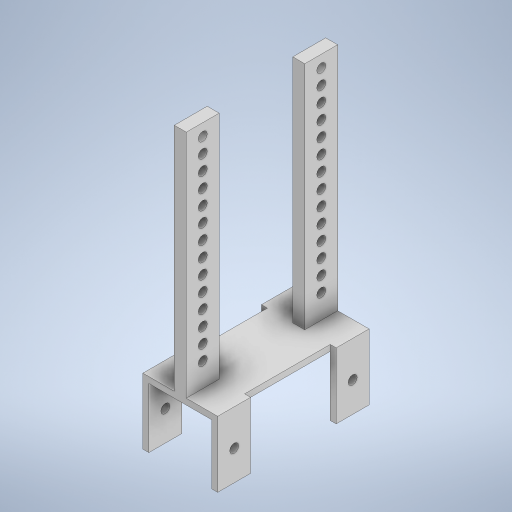
# Autodesk Inventor part: catcher_2ea
Saved by Autodesk Inventor 2024 (Build 280153000, 153)
## iProperties
Created: 2024-07-10
Part Number: catcher_2ea
Material: 일반
Document SubType Name: Modeling
Designer: Gihyeok Na
Density: 1 g/cm^3
Appearance: 기본값
Author: Gihyeok Na
Autodesk Inventor part; units mm, degrees
ref_plane "YZ Plane" through (0, 0, 0) normal (1, 0, 0) x (0, 1, 0)
ref_plane "XZ Plane" through (0, 0, 0) normal (0, 1, 0) x (-1, 0, 0)
ref_plane "XY Plane" through (0, 0, 0) normal (0, 0, 1) x (1, 0, 0)
sketch "스케치4" plane through (0, 0, 0) normal (0, 1, 0) x (-1, 0, 0)
  line L0 (-2, 5.5) -> (-2, -5.5)
  line L1 (-2, -5.5) -> (2, -5.5)
  line L2 (2, -5.5) -> (2, 5.5)
  line L3 (2, 5.5) -> (-2, 5.5)
  line L4 (-2, 5.5) -> (2, -5.5) construction
  line L5 (-2, -5.5) -> (2, 5.5) construction
  line L6 (15.7602, 19.8) -> (-23.0581, 19.8) construction
  line L7 (-2, 34.1) -> (-2, 45.1)
  line L8 (-2, 45.1) -> (2, 45.1)
  line L9 (2, 45.1) -> (2, 34.1)
  line L10 (2, 34.1) -> (-2, 34.1)
  line L11 (-2, 34.1) -> (2, 45.1) construction
  line L12 (-2, 45.1) -> (2, 34.1) construction
  point P0 (0, 0)
  point P1 (0, 0)
  point P2 (0, 39.6)
  point P3 (0, 39.6)
  dimension "d12" = 11
  dimension "d13" = 4
  dimension "d42" = 19.8
  constraints: 26 end point, 6 symmetric about line, 5 midpoint, 2 parallel, 1 horizontal, 1 perpendicular, 1 vertical
  measures "d12" distance of L0.start L0.end
  measures "d13" distance of L1.end L0.end
  measures "d42" distance from line of point (0, 0) L6
extrude "돌출3" add sketch "스케치4" along normal blind 77
sketch "스케치5" plane through (0, 0, 0) normal (0, -1, 0) x (1, 0, 0)
  line L0 (-10.5, -5.5) -> (10.5, -5.5)
  line L1 (10.5, -5.5) -> (10.5, 5.5)
  line L2 (10.5, 5.5) -> (-10.5, 5.5)
  line L3 (-10.5, 5.5) -> (-10.5, -5.5)
  line L4 (-10.5, -5.5) -> (10.5, 5.5) construction
  line L5 (10.5, -5.5) -> (-10.5, 5.5) construction
  line L6 (0, 5.5) -> (0, -5.5) construction
  line L7 (10.5, 5.5) -> (12.5, 5.5)
  line L8 (12.5, 5.5) -> (12.5, -5.5)
  line L9 (12.5, -5.5) -> (10.5, -5.5)
  line L10 (-10.5, 5.5) -> (-12.5, 5.5)
  line L11 (-12.5, 5.5) -> (-12.5, -5.5)
  line L12 (-12.5, -5.5) -> (-10.5, -5.5)
  line L13 (-22.4262, 19.8) -> (40.7349, 19.8) construction
  line L14 (-10.5, 45.1) -> (10.5, 45.1)
  line L15 (10.5, 45.1) -> (10.5, 34.1)
  line L16 (10.5, 34.1) -> (-10.5, 34.1)
  line L17 (-10.5, 34.1) -> (-10.5, 45.1)
  line L18 (-10.5, 45.1) -> (10.5, 34.1) construction
  line L19 (10.5, 45.1) -> (-10.5, 34.1) construction
  line L20 (0, 34.1) -> (0, 45.1) construction
  line L21 (10.5, 34.1) -> (12.5, 34.1)
  line L22 (12.5, 34.1) -> (12.5, 45.1)
  line L23 (12.5, 45.1) -> (10.5, 45.1)
  line L24 (-10.5, 34.1) -> (-12.5, 34.1)
  line L25 (-12.5, 34.1) -> (-12.5, 45.1)
  line L26 (-12.5, 45.1) -> (-10.5, 45.1)
  point P0 (0, 0)
  point P1 (0, 0)
  point P2 (0, 39.6)
  point P3 (0, 39.6)
  dimension "d16" = 21
  dimension "d17" = 11
  dimension "d18" = 2
  dimension "d43" = 19.8
  constraints: 54 end point, 14 symmetric about line, 7 midpoint, 3 horizontal, 3 perpendicular, 2 parallel
  measures "d16" distance of L0.start L0.end
  measures "d17" distance of L1.end L0.end
  measures "d18" distance of L1.end L7.end
  measures "d43" distance from line of point (0, 0) L13
extrude "돌출4" add sketch "스케치5" along normal blind 2
extrude "돌출5" add sketch "스케치5" along normal blind 22 contours L12 L11 L10 L3 | L1 L7 L8 L9 | L17 L24 L25 L26 | L23 L22 L21 L15
sketch "스케치6" plane through (-12.5, 0, -5.5) normal (-1, 0, 0) x (0, 0, 1)
  line L0 (11, 0) -> (0, 0) projected
  line L1 (0, 0) -> (0, -22) projected
  line L2 (11, -22) -> (0, -22) projected
  line L3 (11, 0) -> (11, -22) projected
  circle A0 centre (5.5, -12) radius 1.5
  line L4 (25.3, -63.5481) -> (25.3, 115.0897)
  line L5 (11, 0) -> (11, 77) projected
  line L6 (39.6, -22) -> (50.6, -22)
  circle A1 centre (45.1, -12) radius 1.5
  point P0 (5.5, 0)
  point P1 (25.3, 25.7708)
  dimension "d23" = 3
  dimension "d24" = 10
  dimension "d44" = 14.3
  constraints: 4 end point, 3 symmetric about line, 2 centre point, 1 midpoint, 1 vertical, 1 other
  measures "d23" diameter of A0
  measures "d24" distance from line of A0.centre L2
  measures "d44" distance from line of point (25.3, 25.771) L5
extrude "돌출6" cut sketch "스케치6" against normal through all contours A0 | A1
sketch "스케치7" plane through (-2, 77, -5.5) normal (-1, 0, 0) x (0, 0, 1)
  line L0 (0, -77) -> (11, -77) projected
  line L1 (11, -77) -> (11, 0) projected
  line L2 (0, 0) -> (11, 0) projected
  line L3 (0, -77) -> (0, 0) projected
  line L4 (0, -73) -> (11, -73) construction
  line L5 (0, -4) -> (11, -4) construction
  line L6 (0, -69) -> (11, -69) construction
  circle A0 centre (5.5, -4) radius 1.5
  circle A1 centre (5.5, -69) radius 1.5
  line L7 (5.5, -69) -> (5.5, -4) construction
  circle A2 centre (5.5, -64) radius 1.5
  circle A3 centre (5.5, -59) radius 1.5
  circle A4 centre (5.5, -54) radius 1.5
  circle A5 centre (5.5, -49) radius 1.5
  circle A6 centre (5.5, -44) radius 1.5
  circle A7 centre (5.5, -39) radius 1.5
  circle A8 centre (5.5, -34) radius 1.5
  circle A9 centre (5.5, -29) radius 1.5
  circle A10 centre (5.5, -24) radius 1.5
  circle A11 centre (5.5, -19) radius 1.5
  circle A12 centre (5.5, -14) radius 1.5
  circle A13 centre (5.5, -9) radius 1.5
  line L8 (25.3, -134.2838) -> (25.3, 22.0863) construction
  line L9 (50.6, -77) -> (39.6, -77)
  line L10 (39.6, -77) -> (39.6, 0)
  line L11 (50.6, 0) -> (39.6, 0)
  line L12 (50.6, -77) -> (50.6, 0)
  line L13 (50.6, -73) -> (39.6, -73) construction
  line L14 (50.6, -4) -> (39.6, -4) construction
  line L15 (50.6, -69) -> (39.6, -69) construction
  circle A14 centre (45.1, -4) radius 1.5
  circle A15 centre (45.1, -69) radius 1.5
  line L16 (45.1, -69) -> (45.1, -4) construction
  circle A16 centre (45.1, -64) radius 1.5
  circle A17 centre (45.1, -59) radius 1.5
  circle A18 centre (45.1, -54) radius 1.5
  circle A19 centre (45.1, -49) radius 1.5
  circle A20 centre (45.1, -44) radius 1.5
  circle A21 centre (45.1, -39) radius 1.5
  circle A22 centre (45.1, -34) radius 1.5
  circle A23 centre (45.1, -29) radius 1.5
  circle A24 centre (45.1, -24) radius 1.5
  circle A25 centre (45.1, -19) radius 1.5
  circle A26 centre (45.1, -14) radius 1.5
  circle A27 centre (45.1, -9) radius 1.5
  point P0 (5.5, -77)
  point P1 (45.1, -77)
  dimension "d27" = 4
  dimension "d28" = 4
  dimension "d29" = 4
  dimension "d30" = 3
  dimension "d31" = 5.5
  dimension "d32" = 3
  dimension "d35" = 5
  dimension "d45" = 14.3
  constraints: 28 centre point, 26 end point, 25 symmetric about line, 10 point on line, 4 perpendicular, 3 midpoint, 2 vertical, 38 other
  measures "d27" distance between parallel lines of L4 L0
  measures "d28" distance between parallel lines of L5 L2
  measures "d29" distance between parallel lines of L6 L4
  measures "d30" diameter of A0
  measures "d31" distance from line of L3 L7.end
  measures "d32" diameter of A1
  measures "d35" distance of L7.start A2.centre
  measures "d45" distance between parallel lines of L1 L8
extrude "돌출7" cut sketch "스케치7" against normal through all contours A0 | A1 | A2 | A3 | A4 | A5 | A6 | A7 | A8 | A9 | A10 | A11 | A12 | A13 | A14 | A15 | A16 | A17 | A18 | A19 | A20 | A21 | A22 | A23 | A24 | A25 | A26 | A27
sketch "스케치9" plane through (2, 77, 34.1) normal (0, 0, -1) x (-1, 0, 0)
  line L0 (-8.5, -79) -> (-8.5, -77)
  line L1 (-10.5, -77) -> (0, -77) projected
  line L2 (-8.5, -79) -> (12.5, -79) projected
  line L3 (12.5, -79) -> (12.5, -77)
  line L4 (14.5, -77) -> (4, -77) projected
  line L5 (14.5, -77) -> (4, -77) projected
  line L6 (4, -77) -> (4, 0) projected
  line L7 (0, 0) -> (4, 0) projected
  line L8 (0, -77) -> (0, 0) projected
  line L9 (0, -77) -> (-10.5, -77) projected
  line L10 (-10.5, -77) -> (-10.5, -99) projected
  line L11 (-8.5, -99) -> (-10.5, -99) projected
  line L12 (-8.5, -79) -> (-8.5, -99) projected
  line L13 (12.5, -79) -> (-8.5, -79) projected
  line L14 (12.5, -79) -> (12.5, -99) projected
  line L15 (14.5, -99) -> (12.5, -99) projected
  line L16 (14.5, -77) -> (14.5, -99) projected
  line L17 (0, -77) -> (4, -77)
  point P0 (2, -77)
  point P1 (4, -77)
  constraints: 6 end point, 2 point on line, 1 collinear, 1 parallel, 1 vertical
extrude "돌출8" add sketch "스케치9" along normal up to surface (28.6 mm away) contours L0 L1 L17 L4 L3 L2
